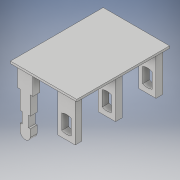
# Autodesk Inventor part: M211LCW01-terminals
Saved by Autodesk Inventor 2019 (Build 230136000, 136)
## iProperties
Created: 2022-08-22
Part Number: M211LCW01-terminals
Material: Generic
Catalog Web Link: www.cadenas.de
Description: M2100 Series LED Tipped Actuators - terminals-
Vendor: NKKSWITCHES
Document SubType Name: Modeling
Designer: psAdmin
Manufacturer: NKKSWITCHES
Mass: 0.0529722 g
Surface Area: 3.15757 cm^2
Volume: 0.0529722 cm^3
Density: 1 g/cm^3
Appearance: PSOLRGB-191-191-191
Category: PARTsolutions
Company: NKKSWITCHES
Title: M211LCW01-terminals
Author: Cadenas PARTsolutions
PSOL_IDENT_0: {$CADENAS_DATA/23d-libs/nkkswitches/toggle/m2100/parts/m2100_terminals.prj},241 {VTYP=3D},{NB=M211LC
PSOL_IDENT_1: W01-terminals},{LINA=M211LCW01-terminals},{NN=M2100 Series LED Tipped Actuators - terminals},{DATE=0
PSOL_IDENT_2: 2.08.2022 07:27:13},{GEOMDATE=23.04.2009 12:08:00},{VERSION=},{LINEID=10},{WBVAR=PLS,LCAT,LEDCLR,CMR
PSOL_IDENT_3: T,TMT},{WBNUMERIC=}  {NB=M211LCW01-terminals},{LINA=M211LCW01-terminals},{KT=DUMMY},{PN=M211LCW01},{
PSOL_IDENT_4: SRS=M21},{PLS=1},{LCAT=L},{LCAT1= 'L','L - Isolated (Toggle)','T','T - Synchronous (Toggle)','R','R
PSOL_IDENT_5: - Isolated (Rocker)','N','N - Synchronous (Rocker)','P','P - Isolated (Paddle)','J','J - Synchronous
PSOL_IDENT_6: (Paddle)' },{LEDCLR=C},{CMRT=W},{TRMNLSCLR=0.75,0.75,0.75,0.00},{TMT=01},{TMT1= '01','01 - Solder L
PSOL_IDENT_7: ug with Threaded Bushing','02','02 - Quick Connect with Threaded Bushing','03','03 - Straight PC wit
PSOL_IDENT_8: h Threaded Bushing' }
NB: M211LCW01-terminals
NN: M2100 Series LED Tipped Actuators - terminals
NBSYN: $PN.-terminals
LINA: M211LCW01-terminals
CATALOG: NKK Switches
PN: M211LCW01
SRS: M21
PLS: 1 - SPDT
LCAT: L - Isolated (Toggle)
LEDCLR: C - Red (Single Color)
CMRT: W - Silver; Rated 6A @ 125V AC
TMT: 01 - Solder Lug with Threaded Bushing
SUPPLIER: NKKSWITCHES
ARTICLENO: M211LCW01-terminals
BOMINFO: M211LCW01-terminals
CREATOR: CADENAS GmbH
Autodesk Inventor part; units mm, degrees
sketch "Sketch_1" plane through (0, 0.762, 0) normal (0, 1, 0) x (1, 0, 0)
  line L0 (-6.096, 6.096) -> (-6.096, -6.096)
  line L1 (-6.096, -6.096) -> (6.096, -6.096)
  line L2 (6.096, -6.096) -> (6.096, 6.096)
  line L3 (6.096, 6.096) -> (-6.096, 6.096)
  constraints: 8 end point
extrude "Extrusion1" add sketch "Sketch_1" along normal blind 0.254
sketch "Sketch_2" plane through (0, 0, 0) normal (0, 0, 1) x (1, 0, 0)
  line L0 (1.397, -3.9878) -> (3.4036, -3.9878)
  line L1 (3.4036, -3.9878) -> (3.4036, 0.762)
  line L2 (3.4036, 0.762) -> (1.397, 0.762)
  line L3 (1.397, 0.762) -> (1.397, -3.9878)
  line L4 (1.8542, -1.5367) -> (1.8542, -3.2893)
  arc A0 (1.8542, -3.2893) -> (2.9464, -3.2893) centre (2.4003, -2.1787) ccw
  line L5 (2.9464, -3.2893) -> (2.9464, -1.5367)
  arc A1 (2.9464, -1.5367) -> (1.8542, -1.5367) centre (2.4003, -2.6473) ccw
  constraints: 12 end point, 4 point on circle, 2 centre point
extrude "Extrusion2" add sketch "Sketch_2" along normal mid plane 10.1854
sketch "Sketch_3" plane through (0, 0, 0) normal (0, 0, 1) x (1, 0, 0)
  line L0 (-3.2893, -1.5494) -> (-2.9845, -1.5494)
  line L1 (-2.9845, -1.5494) -> (-2.9845, -3.6957)
  line L2 (-2.9845, -3.6957) -> (-2.7813, -3.6957)
  line L3 (-2.7813, -3.6957) -> (-2.7813, -4.9657)
  line L4 (-2.7813, -4.9657) -> (-2.9845, -4.9657)
  line L5 (-2.9845, -4.9657) -> (-2.9845, -5.842)
  arc A0 (-2.9845, -5.842) -> (-1.8161, -5.842) centre (-2.4003, -5.7601) ccw
  line L6 (-1.8161, -5.842) -> (-1.8161, -4.9657)
  line L7 (-1.8161, -4.9657) -> (-2.0193, -4.9657)
  line L8 (-2.0193, -4.9657) -> (-2.0193, -3.6957)
  line L9 (-2.0193, -3.6957) -> (-1.8161, -3.6957)
  line L10 (-1.8161, -3.6957) -> (-1.8161, -1.5494)
  line L11 (-1.8161, -1.5494) -> (-1.5113, -1.5494)
  line L12 (-1.5113, -1.5494) -> (-1.5113, 0.762)
  line L13 (-1.5113, 0.762) -> (-3.2893, 0.762)
  line L14 (-3.2893, 0.762) -> (-3.2893, -1.5494)
  constraints: 30 end point, 2 point on circle, 1 centre point
extrude "Extrusion3" add sketch "Sketch_3" along normal mid plane 10.1854
sketch "Sketch_4" plane through (0, 0, 0) normal (1, 0, 0) x (0, 1, 0)
  line L0 (-7.1882, 5.9756) -> (-7.1882, -5.9196)
  line L1 (-7.1882, -5.9196) -> (0.762, -5.9196)
  line L2 (0.762, -5.9196) -> (0.762, -5.0927)
  line L3 (0.762, -5.0927) -> (-6.35, -5.0927)
  line L4 (-6.35, -5.0927) -> (-6.35, -4.3053)
  line L5 (-6.35, -4.3053) -> (0.762, -4.3053)
  line L6 (0.762, -4.3053) -> (0.762, -0.3937)
  line L7 (0.762, -0.3937) -> (-6.35, -0.3937)
  line L8 (-6.35, -0.3937) -> (-6.35, 0.3937)
  line L9 (-6.35, 0.3937) -> (0.762, 0.3937)
  line L10 (0.762, 0.3937) -> (0.762, 4.3053)
  line L11 (0.762, 4.3053) -> (-6.35, 4.3053)
  line L12 (-6.35, 4.3053) -> (-6.35, 5.0927)
  line L13 (-6.35, 5.0927) -> (0.762, 5.0927)
  line L14 (0.762, 5.0927) -> (0.762, 5.9756)
  line L15 (0.762, 5.9756) -> (-7.1882, 5.9756)
  constraints: 32 end point
extrude "Extrusion4" cut sketch "Sketch_4" along normal mid plane 10.16
sketch "Sketch_19" plane through (0, 0.762, 0) normal (0, 1, 0) x (1, 0, 0)
  line L0 (-6.096, 6.096) -> (-6.096, -6.096)
  line L1 (-6.096, -6.096) -> (6.096, -6.096)
  line L2 (6.096, -6.096) -> (6.096, 6.096)
  line L3 (6.096, 6.096) -> (-6.096, 6.096)
  line L4 (-3.81, -5.4076) -> (3.9067, -5.4076)
  line L5 (3.9067, -5.4076) -> (3.9067, 5.3855)
  line L6 (3.9067, 5.3855) -> (-3.81, 5.3855)
  line L7 (-3.81, 5.3855) -> (-3.81, -5.4076)
  constraints: 16 end point
extrude "Extrusion5" cut sketch "Sketch_19" along normal blind 2.54
sketch "Sketch_24" plane through (0, 0, 0) normal (0, 0, 1) x (1, 0, 0)
  line L0 (-8.7503, -7.62) -> (-1.2573, -7.62)
  line L1 (-1.2573, -7.62) -> (-1.2573, 0.762)
  line L2 (-1.2573, 0.762) -> (-8.7503, 0.762)
  line L3 (-8.7503, 0.762) -> (-8.7503, -7.62)
  constraints: 8 end point
extrude "Extrusion6" cut sketch "Sketch_24" along normal mid plane 2.54
ref_plane "terminal_to_body_XY" through (0, 0, 0) normal (0, 1, 0) x (1, 0, 0)
ref_plane "terminal_to_body_YZ" through (0, 0, 0) normal (1, 0, 0) x (0, 0, -1)
ref_plane "terminal_to_body_ZX" through (0, 0, 0) normal (0, 0, -1) x (0, 1, 0)
body "Solid1"
